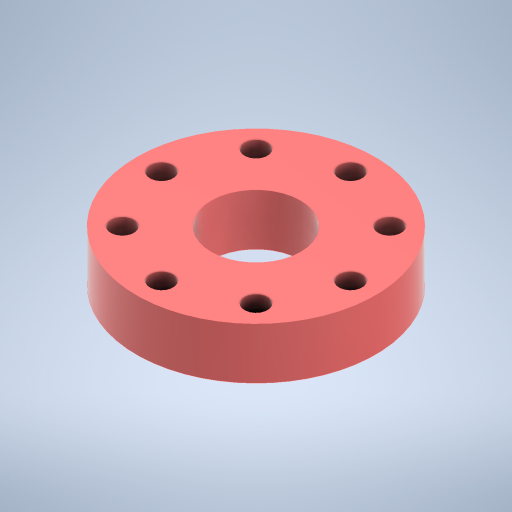
# Autodesk Inventor part: long_horn1
Saved by Autodesk Inventor 2024 (Build 280153000, 153)
## iProperties
Created: 2024-09-08
Part Number: long_horn1
Material: PMMA 플라스틱
Document SubType Name: Modeling
Designer: jmha0
Density: 1.188 g/cm^3
Appearance: 매끄러움 - 빨간색
Author: jmha0
Autodesk Inventor part; units mm, degrees
ref_plane "YZ Plane" through (0, 0, 0) normal (1, 0, 0) x (0, 1, 0)
ref_plane "XZ Plane" through (0, 0, 0) normal (0, 1, 0) x (-1, 0, 0)
ref_plane "XY Plane" through (0, 0, 0) normal (0, 0, 1) x (1, 0, 0)
sketch "스케치1" plane through (0, 0, 0) normal (0, 1, 0) x (-1, 0, 0)
  circle A0 centre (13.7314, -40.8752) radius 1.55
  circle A1 centre (29.2877, -40.8752) radius 1.55
  circle A2 centre (29.2877, -25.3189) radius 1.55
  circle A3 centre (13.7314, -25.3189) radius 1.55
  circle A4 centre (21.5095, -33.0971) radius 13.9
  circle A5 centre (21.5095, -22.0971) radius 1.55
  circle A6 centre (32.5095, -33.0971) radius 1.55
  circle A7 centre (21.5095, -44.0971) radius 1.55
  circle A8 centre (10.5095, -33.0971) radius 1.55
  circle A9 centre (21.5095, -33.0971) radius 5.2
  circle A10 centre (29.2877, -40.8752) radius 1.35
  circle A11 centre (21.5095, -44.0971) radius 1.35
  circle A12 centre (13.7314, -40.8752) radius 1.35
  circle A13 centre (10.5095, -33.0971) radius 1.35
  circle A14 centre (13.7314, -25.3189) radius 1.35
  circle A15 centre (21.5095, -22.0971) radius 1.35
  circle A16 centre (29.2877, -25.3189) radius 1.35
  circle A17 centre (32.5095, -33.0971) radius 1.35
  point P0 (0, 0)
  point P1 (21.5095, -33.0971)
  dimension "d3" = 2.7
  dimension "d4" = 2.7
  dimension "d5" = 2.7
  dimension "d6" = 2.7
  dimension "d7" = 2.7
  dimension "d8" = 2.7
  dimension "d9" = 2.7
  dimension "d10" = 2.7
  constraints: 18 centre point, 8 coincident
  measures "d3" diameter of A10
  measures "d4" diameter of A11
  measures "d5" diameter of A12
  measures "d6" diameter of A13
  measures "d7" diameter of A14
  measures "d8" diameter of A15
  measures "d9" diameter of A16
  measures "d10" diameter of A17
extrude "돌출1" add sketch "스케치1" along normal blind 6 contours A0 | A1 | A2 | A3 | A4 | A5 | A6 | A7 | A8
